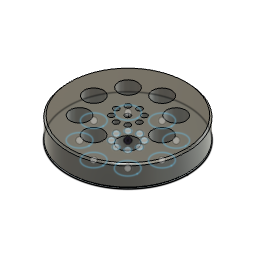
Wheel v3 (Autodesk Fusion 360 design; units mm, degrees)
Autodesk Fusion 360 part; units mm, degrees
sketch "Sketch1" plane through (0, 0, 0) normal (0, 1, 0) x (1, 0, 0) in component "Wheel"
  circle A0 centre (0, 0) radius 55
  circle A1 centre (0.0855, 31.5759) radius 8.75
  circle A2 centre (-22.2671, 22.388) radius 8.75
  circle A3 centre (-31.5759, 0.0855) radius 8.75
  circle A4 centre (-22.388, -22.2671) radius 8.75
  circle A5 centre (-0.0855, -31.5759) radius 8.75
  circle A6 centre (22.2671, -22.388) radius 8.75
  circle A7 centre (31.5759, -0.0855) radius 8.75
  circle A8 centre (22.388, 22.2671) radius 8.75
  line L0 (-1.4465, 2.1) -> (1.4465, 2.1)
  arc A9 (-1.4465, 2.1) -> (1.4465, 2.1) centre (0, 0) ccw
  circle A10 centre (-0.0855, -10.7672) radius 2.55
  circle A11 centre (7.5531, -7.674) radius 2.55
  circle A12 centre (10.7672, -0.0855) radius 2.55
  circle A13 centre (7.674, 7.5531) radius 2.55
  circle A14 centre (0.0855, 10.7672) radius 2.55
  circle A15 centre (-7.5531, 7.674) radius 2.55
  circle A16 centre (-10.7672, 0.0855) radius 2.55
  circle A17 centre (-7.674, -7.5531) radius 2.55
  dimension "d1" = 110
  dimension "d5" = 5.1
  dimension "d6" = 17.5
  dimension "d8" = 360
  dimension "d9" = 2.1
  dimension "d12" = 5.1
  dimension "d14" = 360
  constraint coincident A0.centre A9.centre
  constraint horizontal L0
  constraint vertical A5.centre A10.centre
  measures "d1" diameter of A0
  measures "d5" diameter of A9
  measures "d6" diameter of A1
  measures "d9" distance of A0.centre L0
  measures "d12" diameter of A10
extrude "Extrude2" add sketch "Sketch1" along normal blind 20 in component "Wheel"
fillet "Fillet1" radius 1.5 tangency weight 0.16917 2 edges at (-51.278, 20, 19.8888) (-51.278, 0, 19.8888) in component "Wheel"
component "Wheel" placed x (1, 0, 0) y (0, 1, 0) z (0, 0, 1) at (0, 0, 0)
equation "d1 = ( 55 * 2 ) * 1 mm"
